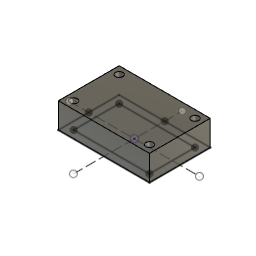
DashLogger v1 (Autodesk Fusion 360 design; units mm, degrees)
Autodesk Fusion 360 part; units mm, degrees
sketch "Skizze1" plane through (0, 0, 0) normal (0, 0, 1) x (1, 0, 0)
  line L0 (-90, -60) -> (90, -60)
  line L1 (90, -60) -> (90, 60)
  line L2 (90, 60) -> (-90, 60)
  line L3 (-90, 60) -> (-90, -60)
  line L4 (0, -120.4862) -> (0, 94.8054) construction
  line L5 (-128.125, 0) -> (128.8109, 0) construction
  line L6 (-75, 45) -> (75, 45)
  line L7 (75, 45) -> (75, -45)
  line L8 (75, -45) -> (-75, -45)
  line L9 (-75, -45) -> (-75, 45)
  point P0 (0, 60)
  point P1 (-90, 0)
  point P2 (-75, 45)
  point P3 (75, 45)
  point P4 (75, -45)
  point P5 (-75, -45)
  dimension "d1" = 120
  dimension "d2" = 180
  dimension "d3" = 15
  dimension "d4" = 15
  dimension "d5" = 15
  dimension "d6" = 15
  constraint horizontal L0
  constraint vertical L1
  constraint horizontal L2
  constraint vertical L3
  constraint perpendicular L2 L4
  constraint coincident origin L4
  constraint midpoint L2 P0
  constraint coincident L4 P0
  constraint horizontal L5
  constraint coincident origin L5
  constraint midpoint L3 P1
  constraint coincident L5 P1
  constraint horizontal L6
  constraint vertical L7
  constraint horizontal L8
  constraint vertical L9
  constraint coincident P2 L6.start
  constraint coincident P3 L6.end
  constraint coincident P4 L7.end
  constraint coincident P5 L8.end
  measures "d1" distance of L0.end L1.end
  measures "d2" distance of L1.end L2.end
  measures "d3" distance of L1 L7
  measures "d4" distance of L2 L6
  measures "d5" distance of L3 L9
  measures "d6" distance of L0 L8
extrude "Extrusion1" add sketch "Skizze1" along normal blind 50 contours L0 L1 L2 L3 | L6 L7 L8 L9
sketch "Skizze2" plane through (0, 0, 50) normal (0, 0, 1) x (-1, 0, 0)
  line L0 (90, -60) -> (90, 60)
  line L1 (90, 60) -> (-90, 60)
  line L2 (-90, 60) -> (-90, -60)
  line L3 (-90, -60) -> (90, -60)
  point P0 (-75, 45)
  point P1 (-75, -45)
  point P2 (75, -45)
  point P3 (75, 45)
hole "Bohrung1" at (-75, 45, 50) at (-75, -45, 50) at (75, -45, 50) at (75, 45, 50) direction (0, 0, -1) diameter 6.6 depth 50 tip angle 180 counterbore diameter 14.55 counterbore depth 40
